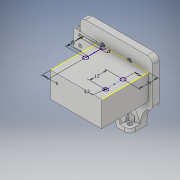
# Autodesk Inventor part: x-carriage-v2
Saved by Autodesk Inventor 2018 (Build 220112000, 112)
## iProperties
Created: 2017-10-14
Part Number: x-carriage-v2
Material: Generic
Document SubType Name: Modeling
Designer: Jurjen
Density: 1 g/cm^3
Appearance: Default
Author: Jurjen
Autodesk Inventor part; units mm, degrees
ref_plane "YZ Plane" through (0, 0, 0) normal (1, 0, 0) x (0, 1, 0)
ref_plane "XZ Plane" through (0, 0, 0) normal (0, 1, 0) x (-1, 0, 0)
ref_plane "XY Plane" through (0, 0, 0) normal (0, 0, 1) x (1, 0, 0)
sketch "Sketch1" plane through (0, 0, 0) normal (0, 0, 1) x (1, 0, 0)
  line L0 (-27, 20) -> (27, 20)
  line L1 (27, 20) -> (27, -15)
  line L2 (27, -15) -> (-27, -15)
  line L3 (-27, -15) -> (-27, 20)
  point P0 (0, 0)
  point P1 (0, 20)
  point P2 (-27, 2.5)
  dimension "d0" = 54
  dimension "d69" = 20
  dimension "d70" = 15
  constraints: 8 end point, 2 midpoint, 2 parallel, 1 horizontal, 1 perpendicular, 1 vertical alignment
  measures "d0" distance between parallel lines of L1 L3
  measures "d69" distance from line of L0 point (0, 0)
  measures "d70" distance from line of point (0, 0) L2
extrude "Extrusion1" add sketch "Sketch1" along normal mid plane 5
sketch "Sketch2" plane through (0, 0, 2.5) normal (0, 0, 1) x (1, 0, 0)
  circle A0 centre (10, 10) radius 1.6
  circle A1 centre (-10, 10) radius 1.6
  circle A2 centre (-10, -10) radius 1.6
  circle A3 centre (10, -10) radius 1.6
  line L0 (-10, 10) -> (10, 10) construction
  line L1 (-10, -10) -> (-10, 10) construction
  point P0 (0, 0)
  point P1 (0, 10)
  point P2 (-10, 0)
  dimension "d4" = 20
  dimension "d5" = 20
  dimension "d6" = 3.2
  constraints: 4 centre point, 4 end point, 3 equal radius, 3 horizontal alignment, 3 vertical alignment, 2 midpoint, 1 horizontal, 1 vertical
  measures "d4" distance of L0.end L0.start
  measures "d5" distance of L1.start L0.start
  measures "d6" diameter of A1
extrude "Extrusion2" cut sketch "Sketch2" against normal up to next
fillet "Fillet1" radius 4 4 edges at (-27, 20, 0) (-27, -15, 0) (27, -15, 0) (27, 20, 0)
sketch "Sketch3" plane through (0, 0, 2.5) normal (0, 0, 1) x (1, 0, 0)
  line L0 (-23, -15) -> (23, -15) projected
  arc A0 (8.05, -30) -> (-8.05, -30) centre (0, -30) ccw
  line L1 (18.05, -30) -> (8.05, -30)
  arc A1 (23, -15) -> (18.05, -30) centre (35.5063, -27.4438) ccw
  line L2 (0, -30) -> (0, 0) construction
  line L3 (-18.05, -30) -> (-8.05, -30)
  arc A2 (-18.05, -30) -> (-23, -15) centre (-35.5063, -27.4438) ccw
  dimension "d10" = 30
  dimension "d12" = 10
  dimension "d13" = 16.1
  constraints: 6 end point, 6 point on circle, 3 centre point, 3 symmetric about line, 1 horizontal, 1 horizontal alignment, 1 vertical, 1 vertical alignment, 1 other
  measures "d10" distance of L2.start L2.end
  measures "d12" distance of L1.start L1.end
  measures "d13" diameter of A0
extrude "Extrusion3" add sketch "Sketch3" against normal up to surface (5 mm away)
sketch "Sketch4" plane through (0, 0, 2.5) normal (0, 0, 1) x (1, 0, 0)
  arc A0 (8.05, -30) -> (-8.05, -30) centre (0, -30) ccw projected
  arc A1 (6.15, -30) -> (-6.15, -30) centre (0, -30) ccw
  line L0 (-6.15, -30) -> (-18.05, -30)
  arc A2 (-18.05, -30) -> (-23, -15) centre (-35.5063, -27.4438) ccw projected
  line L1 (18.05, -30) -> (8.05, -30) projected
  line L2 (18.05, -30) -> (6.15, -30)
  arc A3 (8.05, -30) -> (-8.05, -30) centre (0, -30) ccw
  point P0 (0, 0)
  dimension "d16" = 12.3
  constraints: 6 point on circle, 4 end point, 2 centre point, 2 coincident, 2 point on line, 1 collinear, 1 horizontal alignment
  measures "d16" diameter of A1
extrude "Extrusion4" add sketch "Sketch4" along normal blind 3.8 and the other way blind 1.8
sketch "Sketch5" plane through (0, 0, 2.5) normal (0, 0, 1) x (1, 0, 0)
  arc A0 (27, 16) -> (23, 20) centre (23, 16) ccw projected
  line L0 (23, 20) -> (-23, 20) projected
  arc A1 (-23, 20) -> (-27, 16) centre (-23, 16) ccw projected
  line L1 (-27, 16) -> (-27, -11) projected
  arc A2 (-27, -11) -> (-23, -15) centre (-23, -11) ccw projected
  arc A3 (-18.05, -30) -> (-23, -15) centre (-35.5063, -27.4438) ccw projected
  line L2 (-8.05, -30) -> (-18.05, -30) projected
  arc A4 (8.05, -30) -> (-8.05, -30) centre (0, -30) ccw projected
  line L3 (18.05, -30) -> (8.05, -30) projected
  arc A5 (23, -15) -> (18.05, -30) centre (35.5063, -27.4438) ccw projected
  arc A6 (23, -15) -> (27, -11) centre (23, -11) ccw projected
  line L4 (27, -11) -> (27, 16) projected
  circle A7 centre (-10, -10) radius 1.6 projected
  circle A8 centre (10, 10) radius 1.6 projected
  circle A9 centre (-10, 10) radius 1.6 projected
  circle A10 centre (10, -10) radius 1.6 projected
  arc A11 (23, -15) -> (18.05, -30) centre (35.5063, -27.4438) ccw projected
  line L5 (17.8694, -27) -> (7.4701, -27)
  line L6 (-7.4701, -27) -> (-17.8694, -27)
  point P0 (0, 0)
  dimension "d21" = 3
  constraints: 4 end point, 4 point on circle, 2 point on line, 1 horizontal
  measures "d21" distance between parallel lines of L3 L5
extrude "Extrusion5" add sketch "Sketch5" along normal up to surface (3.8 mm away) contours A5 L3 A4 L5 | A4 L2 A3 L6
sketch "Sketch6" plane through (0, 0, 6.3) normal (0, 0, 1) x (1, 0, 0)
  arc A0 (8.05, -30) -> (-8.05, -30) centre (0, -30) ccw projected
  arc A1 (8.05, -30) -> (-8.05, -30) centre (0, -30) ccw
  arc A2 (11.05, -30) -> (-11.05, -30) centre (0, -30) ccw
  arc A3 (6.15, -30) -> (-6.15, -30) centre (0, -30) ccw projected
  line L0 (-6.15, -30) -> (-18.05, -30) projected
  line L1 (-6.15, -30) -> (-18.05, -30)
  line L2 (6.15, -30) -> (12.1947, -30)
  point P0 (0, 0)
  dimension "d24" = 3
  constraints: 6 point on circle, 4 end point, 4 point on line, 2 centre point, 2 coincident, 2 horizontal
  measures "d24" radial gap between concentric circles of A2 A1
extrude "Extrusion6" add sketch "Sketch6" along normal blind 4 contours A0 L0 A2 L2
sketch "Sketch9" plane through (0, 0, 6.3) normal (0, 0, 1) x (1, 0, 0)
  arc A0 (-10.635, -27) -> (-11.05, -30) centre (0, -30) ccw projected
  line L0 (-17.8694, -27) -> (-10.635, -27) projected
  arc A1 (-18.05, -30) -> (-17.8694, -27) centre (-35.5063, -27.4438) ccw projected
  line L1 (-11.05, -30) -> (-18.05, -30) projected
  arc A2 (11.05, -30) -> (10.635, -27) centre (0, -30) ccw projected
  line L2 (11.05, -30) -> (18.05, -30) projected
  arc A3 (17.8694, -27) -> (18.05, -30) centre (35.5063, -27.4438) ccw projected
  line L3 (10.635, -27) -> (17.8694, -27) projected
  point P0 (0, 0)
extrude "Extrusion7" add sketch "Sketch9" along normal up to surface (4 mm away)
sketch "Sketch10" plane through (0, 0, 6.3) normal (0, 0, -1) x (-1, 0, 0)
  line L0 (10.635, -27) -> (7.4701, -27) projected
  arc A0 (10.635, -27) -> (-10.635, -27) centre (0, -30) ccw projected
  line L1 (-7.4701, -27) -> (-10.635, -27) projected
  arc A1 (7.4701, -27) -> (-7.4701, -27) centre (0, -30) ccw projected
  point P0 (0, 0)
extrude "Extrusion8" add sketch "Sketch10" along normal up to surface (3.8 mm away)
chamfer "Chamfer1" distance 5 angle 45 1 edges at (0, -18.95, 2.5)
fillet "Fillet2" radius 4 2 edges at (17.8957, -28.5039, 10.3) (-17.8957, -28.5039, 10.3)
fillet "Fillet3" radius 4 2 edges at (0, -18.95, 7.5) (0, -13.95, 2.5)
sketch "Sketch13" plane through (-18.05, -30, -2.5) normal (0, -1, 0) x (1, 0, 0)
  circle A0 centre (4, 8.8) radius 1.6
  circle A1 centre (32.1, 8.8) radius 1.6
  line L0 (0, 0) -> (0, 8.8) projected
  line L1 (10, 12.8) -> (4.0347, 12.8) projected
  line L2 (36.1, 8.8) -> (36.1, 0) projected
  point P0 (18.05, 2.5)
  dimension "d45" = 3.2
  dimension "d46" = 4
  dimension "d47" = 4
  dimension "d48" = 4
  constraints: 2 centre point, 1 equal radius, 1 horizontal alignment
  measures "d45" diameter of A0
  measures "d46" distance from line of A0.centre L0
  measures "d47" distance from line of L1 A0.centre
  measures "d48" distance from line of A1.centre L2
extrude "Extrusion10" cut sketch "Sketch13" against normal up to next
sketch "Sketch20" plane through (-13.8684, -27, 10.3) normal (0, 1, 0) x (1, 0, 0)
  arc A0 (0.5066, 5.4444) -> (1.2444, 4.7255) centre (-0.1816, 4) ccw projected
  circle A1 centre (-0.1816, 4) radius 1.6 projected
  line L0 (-0.1816, 0.8) -> (-3.0316, 2.3725)
  line L1 (-3.0316, 2.3725) -> (-3.0316, 5.6275)
  line L2 (-3.0316, 5.6275) -> (-0.1816, 7.2)
  line L3 (-0.1816, 7.2) -> (2.6684, 5.6275)
  line L4 (2.6684, 5.6275) -> (2.6684, 2.3725)
  line L5 (2.6684, 2.3725) -> (-0.1816, 0.8)
  point P0 (13.8684, 10.3)
  point P1 (-3.0316, 4)
  dimension "d138" = 5.7
  dimension "d139" = 6.4
  constraints: 12 end point, 3 horizontal alignment, 3 parallel, 2 vertical alignment, 1 equal length, 1 midpoint, 1 vertical, 1 other
  measures "d138" distance between parallel lines of L1 L4
  measures "d139" distance of L2.end L0.start
extrude "Extrusion16" cut sketch "Sketch20" along normal blind 10
mirror "Mirror3" about plane through (0, 0, 0) normal (1, 0, 0) of "Extrusion16"
sketch "Sketch21" plane through (0, 0, 2.5) normal (0, 0, 1) x (1, 0, 0)
  line L0 (-34, 9) -> (-34, -4)
  line L1 (-34, -4) -> (-27, -4)
  line L2 (-27, -11) -> (-27, 16) projected
  line L3 (-34, 9) -> (-27, 9)
  point P0 (0, 0)
  point P1 (-34, 2.5)
  point P2 (-27, 2.5)
  dimension "d142" = 7
  dimension "d143" = 13
  constraints: 6 end point, 2 midpoint, 2 point on line, 1 horizontal alignment, 1 parallel, 1 perpendicular, 1 vertical
  measures "d142" distance between parallel lines of L2 L0
  measures "d143" distance between parallel lines of L1 L3
extrude "Extrusion17" add sketch "Sketch21" against normal up to surface (5 mm away)
sketch "Sketch22" plane through (0, 0, 2.5) normal (0, 0, 1) x (1, 0, 0)
  arc A0 (17.4509, -27) -> (-17.4509, -27) centre (0, -30) ccw projected
  line L0 (17.4509, -27) -> (17.8694, -27) projected
  arc A1 (23, -15) -> (17.8694, -27) centre (35.5063, -27.4438) ccw projected
  arc A2 (23, -15) -> (27, -11) centre (23, -11) ccw projected
  line L1 (27, -11) -> (27, 16) projected
  arc A3 (27, 16) -> (23, 20) centre (23, 16) ccw projected
  line L2 (23, 20) -> (-23, 20) projected
  arc A4 (-23, 20) -> (-27, 16) centre (-23, 16) ccw projected
  line L3 (-27, 16) -> (-27, 9) projected
  line L4 (-27, 9) -> (-34, 9) projected
  line L5 (-34, 9) -> (-34, -4) projected
  line L6 (-34, -4) -> (-27, -4) projected
  line L7 (-27, -4) -> (-27, -11) projected
  arc A5 (-27, -11) -> (-23, -15) centre (-23, -11) ccw projected
  arc A6 (-17.8694, -27) -> (-23, -15) centre (-35.5063, -27.4438) ccw projected
  line L8 (-17.8694, -27) -> (-17.4509, -27) projected
  circle A7 centre (10, -10) radius 1.6 projected
  circle A8 centre (-10, -10) radius 1.6 projected
  circle A9 centre (-28.9, 5.75) radius 1.15
  circle A10 centre (-28.9, -0.75) radius 1.15
  line L9 (-28.9, 5.75) -> (-28.9, -0.75) construction
  point P0 (0, 0)
  point P1 (-28.9, 2.5)
  point P2 (-34, 2.5)
  dimension "d146" = 2.3
  dimension "d147" = 6.5
  dimension "d148" = 5.1
  constraints: 2 centre point, 2 end point, 2 midpoint, 1 equal radius, 1 horizontal alignment, 1 vertical, 1 vertical alignment
  measures "d146" diameter of A9
  measures "d147" distance of L9.end L9.start
  measures "d148" distance from line of L5 L9.start
extrude "Extrusion18" cut sketch "Sketch22" against normal up to next contours A9 | A10
fillet "Fillet8" radius 2 4 edges at (-27, -4, 0) (-34, -4, 0) (-34, 9, 0) (-27, 9, 0)
sketch "Sketch23" plane through (0, 0, 2.5) normal (0, 0, 1) x (1, 0, 0)
  line L0 (-29, 9) -> (-32, 9) projected
  line L1 (-34, 7) -> (-34, -2) projected
  arc A0 (-34, -2) -> (-32, -4) centre (-32, -2) ccw projected
  line L2 (-32, 9) -> (-29, 9)
  line L3 (-32, -4) -> (-32, 9) construction
  line L4 (-34, -2) -> (-34, 7)
  arc A1 (-32, 9) -> (-34, 7) centre (-32, 7) ccw
  line L5 (-16.5, 8.15) -> (-16.5, -4)
  arc A2 (-29, 9) -> (-16.5, 8.15) centre (-16.5, 100.4868) ccw
  arc A3 (-27, -6) -> (-29, -4) centre (-29, -6) ccw projected
  line L6 (-16.5, -4) -> (-32, -4)
  arc A4 (-34, -2) -> (-32, -4) centre (-32, -2) ccw
  line L7 (-32, -4) -> (-29, -4) projected
  point P0 (0, 0)
  point P1 (-16.5, 2.15)
  dimension "d153" = 2
  dimension "d164" = 6
  dimension "d181" = 0.85
  dimension "d183" = 17.5
  constraints: 10 end point, 7 point on circle, 3 centre point, 2 horizontal, 2 point on line, 2 tangent, 1 horizontal alignment, 1 line through centre, 1 vertical alignment
  measures "d153" radius of A1
  measures "d164" distance of L5.start point (-16.5, 2.15)
  measures "d181" vertical distance of L5.start L2.end
  measures "d183" distance between parallel lines of L1 L5
extrude "Extrusion19" cut sketch "Sketch23" against normal blind 2
fillet "Fillet9" radius 2 3 edges at (-22.7644, 8.3627, 2.5) (-16.5, 2.075, 2.5) (-22.75, -4, 2.5)
sketch "Sketch24" plane through (0, 0, 2.5) normal (0, 0, 1) x (1, 0, 0)
  line L0 (-14, 9.5) -> (24, 9.5)
  line L1 (24, 9.5) -> (24, -9.5)
  line L2 (24, -9.5) -> (-14, -9.5)
  line L3 (-14, -9.5) -> (-14, 9.5)
  circle A0 centre (-10, 10) radius 1.6 projected
  circle A1 centre (-10, -10) radius 1.6 projected
  line L4 (-10, 10) -> (-10, -10) construction
  point P0 (0, 0)
  point P1 (-10, 0)
  point P2 (-14, 0)
  dimension "d176" = 38
  dimension "d177" = 14
  dimension "d178" = 19
  constraints: 10 end point, 2 midpoint, 2 parallel, 1 horizontal, 1 horizontal alignment, 1 perpendicular, 1 vertical
  measures "d176" distance between parallel lines of L3 L1
  measures "d177" distance from line of L3 point (0, 0)
  measures "d178" distance between parallel lines of L2 L0
extrude "Extrusion20" add sketch "Sketch24" along normal blind 35 contours L0 A0 L1 L2 A1 L3 | L0 A0 | A1 L2 picked at (-10.2369, 9.1074) picked at (-9.5677, -9.184)
sketch "Sketch25" plane through (8.4801, 9.5, 2.5) normal (0, 1, 0) x (1, 0, 0)
  circle A0 centre (10.5199, -14) radius 1.6
  circle A1 centre (10.5199, -27) radius 1.6
  line L0 (10.5199, -14) -> (10.5199, -27) construction
  line L1 (3.0397, 0) -> (15.5199, 0) projected
  line L2 (15.5199, 0) -> (15.5199, -35) projected
  circle A2 centre (-17.4801, -1) radius 1.6
  circle A3 centre (-17.4801, -14) radius 1.6
  line L3 (-22.4801, 0) -> (-22.4801, -35) projected
  line L4 (-16.9603, 0) -> (0, 0) projected
  line L5 (-17.4801, -1) -> (-17.4801, -14)
  line L6 (-17.4801, -3) -> (-17.4801, -12)
  point P0 (-8.4801, 2.5)
  point P1 (10.5199, -20.5)
  point P2 (-17.4801, -7.5)
  point P3 (-17.4801, -7.5)
  dimension "d184" = 3.2
  dimension "d185" = 13
  dimension "d187" = 14
  dimension "d188" = 5
  dimension "d189" = 13
  dimension "d190" = 5
  dimension "d192" = 9
  dimension "d193" = 3
  constraints: 6 end point, 4 centre point, 3 equal radius, 3 midpoint, 2 point on line, 2 vertical, 1 coincident, 1 vertical alignment
  measures "d184" diameter of A1
  measures "d185" distance of L0.end L0.start
  measures "d187" distance from line of L1 L0.start
  measures "d188" distance from line of L2 L0.start
  measures "d189" distance of L5.start L5.end
  measures "d190" distance from line of L3 L5.end
  measures "d192" distance of L6.start L6.end
  measures "d193" distance from line of L4 L6.start
body "Solid1"
